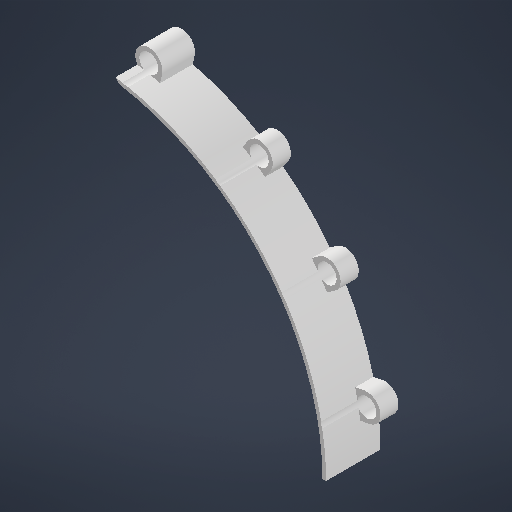
# Autodesk Inventor part: HalfFilterwall3
Saved by Autodesk Inventor 2026 (Build 300175050, 175E)
## iProperties
Created: 2026-05-08
Part Number: HalfFilterwall3
Material: Generic
Document SubType Name: Modeling
Designer: sniel
Density: 1 g/cm^3
Appearance: Default
Author: sniel
Autodesk Inventor part; units mm, degrees
ref_plane "YZ Plane" through (0, 0, 0) normal (1, 0, 0) x (0, 1, 0)
ref_plane "XZ Plane" through (0, 0, 0) normal (0, 1, 0) x (-1, 0, 0)
ref_plane "XY Plane" through (0, 0, 0) normal (0, 0, 1) x (1, 0, 0)
sketch "Sketch2" plane through (0, 0, 0) normal (0, 0, 1) x (1, 0, 0)
  circle A0 centre (138.7343, -109.7729) radius 5.25 projected
  circle A1 centre (116.8119, -56.8475) radius 5.25 projected
  circle A2 centre (26.4627, 2.4988) radius 5.25 projected
  circle A3 centre (79.388, -19.4236) radius 5.25 projected
  line L0 (116.6514, -65.861) -> (120.8614, -63.1603) projected
  arc A4 (120.8614, -63.1603) -> (112.4329, -50.7586) centre (116.8119, -56.8475) ccw projected
  line L1 (112.4329, -50.7586) -> (108.3722, -53.679) projected
  arc A5 (108.3722, -53.679) -> (82.5566, -27.8633) centre (0, -136.2355) ccw projected
  line L2 (82.5566, -27.8633) -> (85.4769, -23.8026) projected
  arc A6 (85.4769, -23.8026) -> (73.0752, -15.3741) centre (79.388, -19.4236) ccw projected
  line L3 (73.0752, -15.3741) -> (70.3746, -19.5842) projected
  arc A7 (70.3746, -19.5842) -> (32.7226, -3.9882) centre (0, -136.2355) ccw projected
  line L4 (32.7226, -3.9882) -> (33.7899, 0.8984) projected
  arc A8 (33.7899, 0.8984) -> (19.0608, 3.7079) centre (26.4627, 2.4988) ccw projected
  line L5 (19.0608, 3.7079) -> (18.2544, -1.2285) projected
  arc A9 (18.2544, -1.2285) -> (0, 0) centre (0, -136.2355) ccw projected
  line L6 (0, 0) -> (0, -2) projected
  arc A10 (134.2355, -136.2355) -> (0, -2) centre (0, -136.2355) ccw projected
  line L7 (134.2355, -136.2355) -> (136.2355, -136.2355) projected
  arc A11 (136.2355, -136.2355) -> (135.007, -117.9811) centre (0, -136.2355) ccw projected
  line L8 (135.007, -117.9811) -> (139.9434, -117.1747) projected
  arc A12 (139.9434, -117.1747) -> (137.1339, -102.4456) centre (138.7343, -109.7729) ccw projected
  line L9 (137.1339, -102.4456) -> (132.2473, -103.5129) projected
  arc A13 (132.2473, -103.5129) -> (116.6514, -65.861) centre (0, -136.2355) ccw projected
  arc A14 (18.2544, -1.2285) -> (-23.9798, -2.127) centre (0, -136.2355) ccw projected
  arc A15 (-27.0685, -2.7162) -> (-23.9798, -2.127) centre (-26.4627, 2.4988) ccw projected
  arc A16 (-27.0685, -2.7162) -> (-75.2721, -22.6828) centre (0, -136.2355) ccw projected
  arc A17 (-77.8727, -24.4502) -> (-75.2721, -22.6828) centre (-79.388, -19.4236) ccw projected
  arc A18 (-77.8727, -24.4502) -> (-111.7853, -58.3628) centre (0, -136.2355) ccw projected
  arc A19 (-113.5527, -60.9634) -> (-111.7853, -58.3628) centre (-116.8119, -56.8475) ccw projected
  arc A20 (-113.5527, -60.9634) -> (-133.5193, -109.1671) centre (0, -136.2355) ccw projected
  arc A21 (-134.1085, -112.2557) -> (-133.5193, -109.1671) centre (-138.7343, -109.7729) ccw projected
  arc A22 (-134.1085, -112.2557) -> (-136.2355, -136.2355) centre (0, -136.2355) ccw projected
  line L10 (-136.2355, -136.2355) -> (-134.2355, -136.2355) projected
  arc A23 (-133.4843, -122.0537) -> (-134.2355, -136.2355) centre (0, -136.2355) ccw projected
  arc A24 (-133.2582, -120.0666) -> (-133.4843, -122.0537) centre (0, -136.2355) ccw projected
  arc A25 (-124.3552, -85.689) -> (-133.2582, -120.0666) centre (0, -136.2355) ccw projected
  arc A26 (-123.5884, -83.8419) -> (-124.3552, -85.689) centre (0, -136.2355) ccw projected
  arc A27 (-90.6982, -37.2759) -> (-123.5884, -83.8419) centre (0, -136.2355) ccw projected
  arc A28 (-89.2138, -35.9356) -> (-90.6982, -37.2759) centre (0, -136.2355) ccw projected
  arc A29 (-24.5369, -4.2616) -> (-89.2138, -35.9356) centre (0, -136.2355) ccw projected
  line L11 (-24.5369, -4.2616) -> (-17.9914, -35.5817) projected
  arc A30 (-24.3732, -35.8597) -> (-17.9914, -35.5817) centre (-22.5679, -3.9107) ccw projected
  arc A31 (-24.3732, -35.8597) -> (-71.7399, -55.1686) centre (-13.0409, -131.4111) ccw projected
  line L12 (-71.7399, -55.1686) -> (-89.2138, -35.9356) projected
  line L13 (-89.2138, -35.9356) -> (-90.6982, -37.2759) projected
  line L14 (-90.6982, -37.2759) -> (-74.6321, -57.4663) projected
  arc A32 (-74.6321, -57.4663) -> (-103.6394, -92.1242) centre (2.2704, -151.2986) ccw projected
  line L15 (-103.6394, -92.1242) -> (-123.5884, -83.8419) projected
  line L16 (-123.5884, -83.8419) -> (-124.3552, -85.689) projected
  line L17 (-124.3552, -85.689) -> (-104.606, -93.8884) projected
  arc A33 (-104.606, -93.8884) -> (-115.4523, -121.9752) centre (2.2704, -151.2986) ccw projected
  line L18 (-115.4523, -121.9752) -> (-133.2582, -120.0666) projected
  line L19 (-133.2582, -120.0666) -> (-133.4843, -122.0537) projected
  line L20 (-133.4843, -122.0537) -> (-115.9197, -123.9199) projected
  arc A34 (-115.9197, -123.9199) -> (-118.1107, -136.2355) centre (2.2704, -151.2986) ccw projected
  line L21 (-118.1107, -136.2355) -> (-115.1005, -136.2355) projected
  arc A35 (-69.7224, -57.3892) -> (-115.1005, -136.2355) centre (4.4084, -152.5347) ccw projected
  arc A36 (-15.6263, -37.1945) -> (-69.7224, -57.3892) centre (-7.9541, -140.298) ccw projected
  arc A37 (-15.6263, -37.1945) -> (18.2544, -1.2285) centre (-20.5393, 1.3748) ccw projected
  circle A38 centre (26.4627, 2.4988) radius 7.5
  point P0 (19.0608, 3.7079)
  point P1 (22.5679, -3.9107)
  constraints: 1 centre point, 1 coincident, 1 tangent
extrude "Extrusion2" add sketch "Sketch2" along normal blind 30 contours A13 L9 A12 L8 A11 L7 A10 A38 L4 A7 L3 A6 L2 A5 L1 A4 L0 | A10 A38 A8
sketch "Sketch3" plane through (0, 0, 30) normal (0, 0, 1) x (1, 0, 0)
  line L0 (32.7226, -3.9882) -> (33.7899, 0.8984) projected
  arc A0 (33.7899, 0.8984) -> (22.5679, -3.9107) centre (26.4627, 2.4988) ccw projected
  arc A1 (134.2355, -136.2355) -> (22.5679, -3.9107) centre (0, -136.2355) ccw projected
  line L1 (134.2355, -136.2355) -> (136.2355, -136.2355) projected
  arc A2 (136.2355, -136.2355) -> (135.007, -117.9811) centre (0, -136.2355) ccw projected
  line L2 (135.007, -117.9811) -> (139.9434, -117.1747) projected
  arc A3 (139.9434, -117.1747) -> (137.1339, -102.4456) centre (138.7343, -109.7729) ccw projected
  line L3 (137.1339, -102.4456) -> (132.2473, -103.5129) projected
  arc A4 (132.2473, -103.5129) -> (116.6514, -65.861) centre (0, -136.2355) ccw projected
  line L4 (116.6514, -65.861) -> (120.8614, -63.1603) projected
  arc A5 (120.8614, -63.1603) -> (112.4329, -50.7586) centre (116.8119, -56.8475) ccw projected
  line L5 (112.4329, -50.7586) -> (108.3722, -53.679) projected
  arc A6 (108.3722, -53.679) -> (82.5566, -27.8633) centre (0, -136.2355) ccw projected
  line L6 (82.5566, -27.8633) -> (85.4769, -23.8026) projected
  arc A7 (85.4769, -23.8026) -> (73.0752, -15.3741) centre (79.388, -19.4236) ccw projected
  line L7 (73.0752, -15.3741) -> (70.3746, -19.5842) projected
  arc A8 (70.3746, -19.5842) -> (32.7226, -3.9882) centre (0, -136.2355) ccw projected
  circle A9 centre (26.4627, 2.4988) radius 5.25 projected
  circle A10 centre (79.388, -19.4236) radius 5.25 projected
  circle A11 centre (116.8119, -56.8475) radius 5.25 projected
  circle A12 centre (138.7343, -109.7729) radius 5.25 projected
  circle A13 centre (0, -136.2355) radius 136.2355
  point P0 (0, 0)
  point P1 (133.5193, -109.1671)
  point P2 (134.1085, -112.2557)
  point P3 (135.007, -117.9811)
  point P4 (111.7853, -58.3628)
  point P5 (113.5527, -60.9634)
  point P6 (116.6514, -65.861)
  point P7 (27.0685, -2.7162)
  point P8 (20.1131, -1.4929)
  point P9 (23.9798, -2.127)
  point P10 (75.2721, -22.6828)
  point P11 (77.8727, -24.4502)
  point P12 (82.5566, -27.8633)
  constraints: 1 coincident, 3 other
extrude "Extrusion3" cut sketch "Sketch3" against normal blind 20 contours A13 A9 A0 L0 | L7 A7 L6 A13 A10 | A13 A12 L3 A3 L2 | L5 A5 L4 A13 A11
sketch "Sketch4" plane through (0, 0, 10) normal (0, 0, 1) x (1, 0, 0)
  line L0 (33.7899, 0.8984) -> (32.7226, -3.9882) projected
  arc A0 (33.7899, 0.8984) -> (20.1131, -1.4929) centre (26.4627, 2.4988) ccw projected
  arc A1 (23.9798, -2.127) -> (20.1131, -1.4929) centre (0, -136.2355) ccw projected
  arc A2 (27.0685, -2.7162) -> (23.9798, -2.127) centre (26.4627, 2.4988) ccw projected
  arc A3 (32.7226, -3.9882) -> (27.0685, -2.7162) centre (0, -136.2355) ccw projected
  point P0 (0, 0)
extrude "Extrusion4" add sketch "Sketch4" along normal blind 8
body "Solid2"
